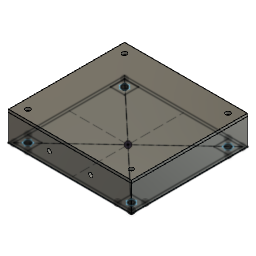
boitepile v1 (Autodesk Fusion 360 design; units mm, degrees)
Autodesk Fusion 360 part; units mm, degrees
sketch "Sketch1" plane through (0, 0, 0) normal (0, 1, 0) x (1, 0, 0)
  line L0 (42.5, 40) -> (-42.5, 40)
  line L1 (-42.5, 40) -> (-42.5, -40)
  line L2 (-42.5, -40) -> (42.5, -40)
  line L3 (42.5, -40) -> (42.5, 40)
  line L4 (42.5, 40) -> (-42.5, -40) construction
  line L5 (-42.5, 40) -> (42.5, -40) construction
  circle A0 centre (-37.5, 35) radius 1.75
  line L6 (-38.1316, 32.3017) -> (-35.479, 33.1038)
  line L7 (-35.479, 33.1038) -> (-34.8474, 35.8022)
  line L8 (-34.8474, 35.8022) -> (-36.8684, 37.6983)
  line L9 (-36.8684, 37.6983) -> (-39.521, 36.8962)
  line L10 (-39.521, 36.8962) -> (-40.1526, 34.1978)
  line L11 (-40.1526, 34.1978) -> (-38.1316, 32.3017)
  line L12 (0, 0) -> (0, 40) construction
  line L13 (0, 0) -> (-42.5, 0) construction
  line L14 (34.8474, 35.8022) -> (36.8684, 37.6983)
  line L15 (36.8684, 37.6983) -> (39.521, 36.8962)
  line L16 (35.479, 33.1038) -> (34.8474, 35.8022)
  line L17 (38.1316, 32.3017) -> (35.479, 33.1038)
  circle A1 centre (37.5, 35) radius 1.75
  line L18 (39.521, 36.8962) -> (40.1526, 34.1978)
  line L19 (40.1526, 34.1978) -> (38.1316, 32.3017)
  line L20 (-40.1526, -34.1978) -> (-38.1316, -32.3017)
  circle A2 centre (-37.5, -35) radius 1.75
  line L21 (-42.5, -40) -> (42.5, 40) construction
  line L22 (-36.8684, -37.6983) -> (-39.521, -36.8962)
  line L23 (-39.521, -36.8962) -> (-40.1526, -34.1978)
  line L24 (-35.479, -33.1038) -> (-34.8474, -35.8022)
  line L25 (-38.1316, -32.3017) -> (-35.479, -33.1038)
  line L26 (-34.8474, -35.8022) -> (-36.8684, -37.6983)
  line L27 (0, 0) -> (0, -40) construction
  line L28 (34.8474, -35.8022) -> (36.8684, -37.6983)
  line L29 (35.479, -33.1038) -> (34.8474, -35.8022)
  line L30 (-42.5, 40) -> (42.5, -40) construction
  line L31 (42.5, -40) -> (-42.5, 40) construction
  line L32 (38.1316, -32.3017) -> (35.479, -33.1038)
  line L33 (36.8684, -37.6983) -> (39.521, -36.8962)
  line L34 (39.521, -36.8962) -> (40.1526, -34.1978)
  line L35 (40.1526, -34.1978) -> (38.1316, -32.3017)
  circle A3 centre (37.5, -35) radius 1.75
  line L36 (-44.5, -42) -> (44.5, -42)
  line L37 (44.5, -42) -> (44.5, 42)
  line L38 (44.5, 42) -> (-44.5, 42)
  line L39 (-44.5, 42) -> (-44.5, -42)
  line L40 (-44.5, -42) -> (44.5, 42) construction
  line L41 (44.5, -42) -> (-44.5, 42) construction
  line L42 (-42.5, 40) -> (-32.5, 40)
  line L43 (-32.5, 40) -> (-32.5, 30)
  line L44 (-32.5, 30) -> (-42.5, 30)
  line L45 (-42.5, 30) -> (-42.5, 40)
  line L46 (32.5, 40) -> (32.5, 30)
  line L47 (32.5, 30) -> (42.5, 30)
  line L48 (-32.5, -40) -> (-32.5, -30)
  line L49 (-32.5, -30) -> (-42.5, -30)
  line L50 (32.5, -30) -> (42.5, -30)
  line L51 (32.5, -40) -> (32.5, -30)
  point P0 (-37.5, 35)
  point P1 (37.5, 35)
  point P2 (-37.5, -35)
  point P3 (37.5, -35)
  dimension "d1" = 85
  dimension "d2" = 80
  dimension "d3" = 3.5
  dimension "d4" = 4.8
  dimension "d5" = 5
  dimension "d6" = 5
  dimension "d13" = 2
  dimension "d14" = 2
  dimension "d17" = 5
  dimension "d18" = 5
  constraint horizontal L0
  constraint perpendicular L0 L1
  constraint parallel L0 L2
  constraint parallel L1 L3
  constraint coincident L4 L12.start
  constraint coincident L5 L12.start
  constraint coincident L12.start L13.start
  constraint coincident P0 A0.centre
  constraint midpoint L0 L12.end
  constraint midpoint L1 L13.end
  constraint symmetric A0 L12 A1
  constraint symmetric L6.start L12 L17.start
  constraint symmetric L6.end L12 L16.start
  constraint symmetric L7.end L12 L14.start
  constraint symmetric L8.end L12 L14.end
  constraint symmetric L9.end L12 L15.end
  constraint symmetric L10.end L12 L18.end
  constraint symmetric P0 L12 P1
  constraint symmetric L0.end L13 L1.end
  constraint symmetric L2.end L13 L0.start
  constraint symmetric A0 L13 A2
  constraint symmetric L6.start L13 L20.end
  constraint symmetric L6.end L13 L24.start
  constraint symmetric L7.end L13 L24.end
  constraint symmetric L8.end L13 L22.start
  constraint symmetric L9.end L13 L22.end
  constraint symmetric L10.end L13 L20.start
  constraint symmetric P0 L13 P2
  constraint midpoint L2 L27.end
  constraint symmetric L0.start L27 L0.end
  constraint symmetric L1.end L27 L2.end
  constraint symmetric L20.start L27 L34.end
  constraint symmetric L22.end L27 L33.end
  constraint symmetric P2 L27 P3
  constraint symmetric L20.end L27 L32.start
  constraint symmetric L22.start L27 L28.end
  constraint symmetric L24.end L27 L28.start
  constraint symmetric L24.start L27 L29.start
  constraint symmetric A2 L27 A3
  constraint horizontal L36
  constraint perpendicular L36 L37
  constraint parallel L36 L38
  constraint parallel L37 L39
  constraint coincident L40 L12.start
  constraint coincident L41 L12.start
  constraint horizontal L42
  constraint vertical L43
  constraint horizontal L44
  constraint vertical L45
  constraint symmetric L12 L42.end L46.start
  constraint symmetric L12 L43.end L46.end
  constraint symmetric L12 L44.end L47.end
  constraint symmetric L13 L42.end L48.start
  constraint symmetric L13 L43.end L48.end
  constraint symmetric L13 L44.end L49.end
  constraint symmetric L27 L48.start L51.start
  constraint symmetric L27 L48.end L50.start
  constraint symmetric L27 L49.end L50.end
  measures "d1" distance of L1.end L2.end
  measures "d2" distance of L0.end L1.end
  measures "d3" diameter of A0
  measures "d4" distance of L7 L10
  measures "d5" distance of L0 P0
  measures "d6" distance of L1 P0
  measures "d13" distance of L1 L39
  measures "d14" distance of L2 L36
  measures "d17" distance of P0 L43
  measures "d18" distance of P0 L44
extrude "Extrude1" add sketch "Sketch1" along normal blind 2 contours L0 L3 L46 L47 | L0 L1 L2 L3 L43 L44 L46 L47 L48 L49 L50 L51 | L0 L1 L42 L43 L44 L45 | L2 L3 L50 L51 | L1 L2 L48 L49 | A0 | L6 L7 L8 L9 L10 L11 | L14 L15 L16 L17 L18 L19 | A1 | L20 L22 L23 L24 L25 L26 | A2 | L28 L29 L32 L33 L34 L35 | A3 | L36 L37 L38 L39 makes body 1
extrude "Extrude2" add sketch "Sketch1" along normal blind 17 contours L0 L3 L46 L47 | L0 L1 L42 L43 L44 L45 | L2 L3 L50 L51 | L1 L2 L48 L49 | L6 L7 L8 L9 L10 L11 | L14 L15 L16 L17 L18 L19 | L20 L22 L23 L24 L25 L26 | L28 L29 L32 L33 L34 L35 | L36 L37 L38 L39 bodies 1
extrude "Extrude3" add sketch "Sketch1" along normal blind 2 from surface at 17 contours L0 L3 L46 L47 | L0 L1 L42 L43 L44 L45 | L2 L3 L50 L51 | L1 L2 L48 L49 | L36 L37 L38 L39 bodies 1
extrude "Extrude4" add sketch "Sketch1" along normal blind 2 from surface at 19 separate body contours L0 L3 L46 L47 | L0 L1 L2 L3 L43 L44 L46 L47 L48 L49 L50 L51 | L0 L1 L42 L43 L44 L45 | L2 L3 L50 L51 | L1 L2 L48 L49 | L6 L7 L8 L9 L10 L11 | L14 L15 L16 L17 L18 L19 | L20 L22 L23 L24 L25 L26 | L28 L29 L32 L33 L34 L35 | L36 L37 L38 L39 makes body 2
extrude "Extrude5" add sketch "Sketch1" along normal blind 2 from surface at 17 contours L0 L1 L2 L3 L43 L44 L46 L47 L48 L49 L50 L51 bodies 2
sketch "Sketch4" plane through (0, 0, 42) normal (0, 0, 1) x (1, 0, 0)
  line L0 (-44.5, 0) -> (44.5, 0)
  line L1 (44.5, 0) -> (44.5, 19)
  line L2 (44.5, 19) -> (-44.5, 19)
  line L3 (-44.5, 19) -> (-44.5, 0)
  line L4 (0, 0) -> (0, 19) construction
  line L5 (44.5, 9.5) -> (-44.5, 9.5) construction
  circle A0 centre (15, 9.5) radius 1.5
  circle A1 centre (-15, 9.5) radius 1.5
  dimension "d29" = 3
  dimension "d30" = 15
  constraint coincident L4.start origin
  constraint midpoint L2 L4.end
  constraint midpoint L1 L5.start
  constraint midpoint L3 L5.end
  constraint coincident L5 A0.centre
  constraint symmetric L4 A0 A1
  measures "d29" diameter of A0
  measures "d30" distance of L4 A0.centre
extrude "Extrude6" cut sketch "Sketch4" against normal blind 12 contours A0 | A1 bodies 1
equation "d1 = long"
equation "d2 = la"
equation "long = 85 mm"
equation "la = 80 mm"
equation "h = 15 mm"
equation "e = 2 mm"
equation "d11 = e"
equation "d13 = e"
equation "d14 = e"
equation "d15 = h + e"
equation "d19 = h + e"
equation "d20 = e"
equation "d22 = h + 2 * e"
equation "d23 = e"
equation "d25 = h + e"
equation "d26 = e"
named bodies: "BoitePileBase", "BoitePileCouvercle"
